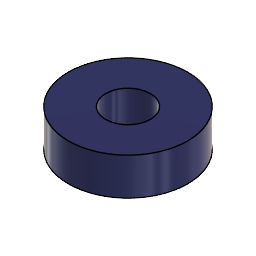
Asembly (Autodesk Fusion 360 archive; units mm, degrees)
design "Guolis 32-20-10"
Autodesk Fusion 360 part; units mm, degrees
sketch "Sketch1" plane through (0, 0, 0) normal (0, 0, 1) x (1, 0, 0)
  circle A0 centre (0, 0) radius 16
  circle A1 centre (0, 0) radius 6
  dimension "d1" = 32
  dimension "d2" = 12
  constraint coincident A0.centre A1.centre
  measures "d1" diameter of A0
  measures "d2" diameter of A1
extrude "Extrude1" add sketch "Sketch1" along normal blind 10

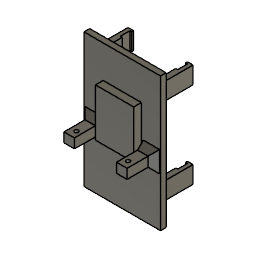
design "Wrist2"
Autodesk Fusion 360 part; units mm, degrees
sketch "Sketch1" plane through (0, 0, 0) normal (0, 1, 0) x (1, 0, 0)
  line L0 (-20, -35) -> (20, -35)
  line L1 (20, -35) -> (20, 35)
  line L2 (20, 35) -> (-20, 35)
  line L3 (-20, 35) -> (-20, -35)
  line L4 (-14.65, -4.5) -> (-12.65, -4.5)
  line L5 (-12.65, -4.5) -> (-12.65, 4.5)
  line L6 (-12.65, 4.5) -> (-14.65, 4.5)
  line L7 (-14.65, 4.5) -> (-14.65, -4.5)
  line L8 (12.65, -4.5) -> (14.65, -4.5)
  line L9 (14.65, -4.5) -> (14.65, 4.5)
  line L10 (14.65, 4.5) -> (12.65, 4.5)
  line L11 (12.65, 4.5) -> (12.65, -4.5)
  line L12 (-12.65, -4.5) -> (-11.65, -4.5)
  line L13 (-11.65, -4.5) -> (-11.65, 4.5)
  line L14 (-11.65, 4.5) -> (-12.65, 4.5)
  line L15 (-12.65, 4.5) -> (-12.65, -4.5)
  line L16 (12.65, -4.5) -> (11.65, -4.5)
  line L17 (11.65, -4.5) -> (11.65, 4.5)
  line L18 (11.65, 4.5) -> (12.65, 4.5)
  line L19 (12.65, 4.5) -> (12.65, -4.5)
  circle A0 centre (0, 0) radius 5
  line L20 (14, 16.5) -> (14, 25.5)
  line L21 (15, 16.5) -> (14, 16.5)
  line L22 (17, 16.5) -> (17, 25.5)
  line L23 (15, 25.5) -> (15, 16.5)
  line L24 (15, 16.5) -> (17, 16.5)
  line L25 (15, 25.5) -> (15, 16.5)
  line L26 (15, -19.5) -> (15, -28.5)
  line L27 (15, -19.5) -> (15, -28.5)
  line L28 (15, -28.5) -> (17, -28.5)
  line L29 (14, -28.5) -> (14, -19.5)
  line L30 (15, -28.5) -> (14, -28.5)
  line L31 (17, -28.5) -> (17, -19.5)
  line L32 (-15, -28.5) -> (-15, -19.5)
  line L33 (-17, -19.5) -> (-17, -28.5)
  line L34 (-15, -28.5) -> (-14, -28.5)
  line L35 (-14, -28.5) -> (-14, -19.5)
  line L36 (-15, -19.5) -> (-17, -19.5)
  line L37 (-15, -19.5) -> (-15, -28.5)
  line L38 (-14, -19.5) -> (-15, -19.5)
  line L39 (-17, -28.5) -> (-15, -28.5)
  line L40 (-15, 16.5) -> (-15, 25.5)
  line L41 (-17, 25.5) -> (-17, 16.5)
  line L42 (-15, 16.5) -> (-14, 16.5)
  line L43 (-14, 16.5) -> (-14, 25.5)
  line L44 (-15, 25.5) -> (-17, 25.5)
  line L45 (-15, 25.5) -> (-15, 16.5)
  line L46 (-14, 25.5) -> (-15, 25.5)
  line L47 (-17, 16.5) -> (-15, 16.5)
  line L48 (17, 25.5) -> (14, 25.5)
  line L49 (17, -19.5) -> (14, -19.5)
  line L50 (12.65, 1.5) -> (14.65, 1.5)
  line L51 (-14.65, 1.5) -> (-12.65, 1.5)
  line L52 (-10, -18) -> (10, -18)
  line L53 (10, -18) -> (10, 7)
  line L54 (10, 7) -> (-10, 7)
  line L55 (-10, 7) -> (-10, -18)
  line L56 (16.5, 1.5) -> (10.5, 1.5)
  line L57 (10.5, 1.5) -> (10.5, 6.5)
  line L58 (10.5, 6.5) -> (16.5, 6.5)
  line L59 (16.5, 6.5) -> (16.5, 1.5)
  line L60 (-10.5, 1.5) -> (-16.5, 1.5)
  line L61 (-16.5, 1.5) -> (-16.5, 6.5)
  line L62 (-16.5, 6.5) -> (-10.5, 6.5)
  line L63 (-10.5, 6.5) -> (-10.5, 1.5)
  dimension "d1" = 40
  dimension "d2" = 70
  dimension "d3" = 20
  dimension "d4" = 35
  dimension "d5" = 9
  dimension "d6" = 2
  dimension "d7" = 4.5
  dimension "d8" = 12.65
  dimension "d9" = 2
  dimension "d10" = 9
  dimension "d11" = 12.65
  dimension "d12" = 4.5
  dimension "d13" = 1
  dimension "d14" = 9
  dimension "d15" = 1
  dimension "d16" = 9
  dimension "d17" = 10
  dimension "d18" = 2
  dimension "d19" = 9
  dimension "d20" = 1
  dimension "d21" = 9
  dimension "d22" = 2
  dimension "d23" = 9
  dimension "d24" = 1
  dimension "d25" = 9
  dimension "d26" = 9
  dimension "d27" = 2
  dimension "d28" = 1
  dimension "d29" = 9
  dimension "d30" = 9
  dimension "d31" = 2
  dimension "d32" = 1
  dimension "d33" = 9
  dimension "d40" = 3
  dimension "d41" = 3
  dimension "d58" = 20
  dimension "d59" = 25
  dimension "d60" = 10
  dimension "d61" = 18
  dimension "d64" = 6
  dimension "d65" = 5
  dimension "d66" = 2.15
  dimension "d67" = 2.15
  dimension "d79" = 3
  dimension "d80" = 3
  dimension "d81" = 3
  dimension "d82" = 3
  constraint horizontal L0
  constraint vertical L1
  constraint horizontal L2
  constraint vertical L3
  constraint horizontal L4
  constraint vertical L5
  constraint horizontal L6
  constraint vertical L7
  constraint horizontal L8
  constraint vertical L9
  constraint horizontal L10
  constraint vertical L11
  constraint horizontal L12
  constraint vertical L13
  constraint horizontal L14
  constraint vertical L15
  constraint horizontal L16
  constraint vertical L17
  constraint horizontal L18
  constraint vertical L19
  constraint coincident A0.centre origin
  constraint horizontal L24
  constraint vertical L22
  constraint vertical L25
  constraint horizontal L21
  constraint vertical L20
  constraint vertical L23
  constraint horizontal L28
  constraint vertical L31
  constraint vertical L27
  constraint horizontal L30
  constraint vertical L29
  constraint vertical L26
  constraint horizontal L39
  constraint vertical L32
  constraint horizontal L36
  constraint vertical L33
  constraint horizontal L34
  constraint vertical L35
  constraint horizontal L38
  constraint vertical L37
  constraint horizontal L47
  constraint vertical L40
  constraint horizontal L44
  constraint vertical L41
  constraint horizontal L42
  constraint vertical L43
  constraint horizontal L46
  constraint vertical L45
  constraint perpendicular L20 L48
  constraint perpendicular L29 L49
  constraint coincident L11 L50.start
  constraint coincident L9 L50.end
  constraint perpendicular L9 L50
  constraint coincident L7 L51.start
  constraint coincident L5 L51.end
  constraint perpendicular L5 L51
  constraint horizontal L52
  constraint vertical L53
  constraint horizontal L54
  constraint vertical L55
  constraint horizontal L56
  constraint vertical L57
  constraint horizontal L58
  constraint vertical L59
  constraint horizontal L60
  constraint vertical L61
  constraint horizontal L62
  constraint vertical L63
  measures "d1" distance of L0.start L0.end
  measures "d2" distance of L0.start L2.end
  measures "d3" horizontal distance of A0.centre L0.start
  measures "d4" vertical distance of A0.centre L0.start
  measures "d5" distance of L4.start L6.end
  measures "d6" distance of L5.end L6.end
  measures "d7" vertical distance of A0.centre L4.end
  measures "d8" distance of A0.centre L5
  measures "d9" distance of L8.start L8.end
  measures "d10" distance of L8.start L10.end
  measures "d11" distance of A0.centre L11
  measures "d12" vertical distance of A0.centre L10.end
  measures "d13" distance of L4.end L12.end
  measures "d14" distance of L4.end L5.end
  measures "d15" distance of L8.start L16.end
  measures "d16" distance of L8.start L10.end
  measures "d17" diameter of A0
  measures "d18" distance of L22.start L21.start
  measures "d19" distance of L21.start L23.start
  measures "d20" distance of L21.start L20.start
  measures "d21" distance of L23.start L21.start
  measures "d22" distance of L28.end L26.end
  measures "d23" distance of L26.start L26.end
  measures "d24" distance of L26.end L29.start
  measures "d25" distance of L26.end L26.start
  measures "d26" distance of L33.end L33.start
  measures "d27" distance of L32.end L33.start
  measures "d28" distance of L32.start L34.end
  measures "d29" distance of L32.start L32.end
  measures "d30" distance of L41.end L41.start
  measures "d31" distance of L40.end L41.start
  measures "d32" distance of L40.start L42.end
  measures "d33" distance of L40.start L40.end
  measures "d40" distance of L10.end L50.start
  measures "d41" distance of L6.end L51.start
  measures "d58" distance of L52.start L52.end
  measures "d59" distance of L52.start L54.end
  measures "d60" distance of A0.centre L55
  measures "d61" distance of A0.centre L52
  measures "d64" distance of L60.start L60.end
  measures "d65" distance of L60.start L62.end
  measures "d66" distance of L19 L57
  measures "d67" distance of L5 L63
  measures "d79" distance of L1 L31
  measures "d80" distance of L3 L33
  measures "d81" distance of L1 L22
  measures "d82" distance of L3 L41
extrude "Extrude1" add sketch "Sketch1" along normal blind 3 contours L0 L1 L2 L3 | L4 L5 L7 L15 L51 L60 | L5 L12 L13 L15 L60 | L6 L7 L13 L14 L60 L61 L62 L63 | L5 L6 L7 L15 L51 L60 | L5 L13 L14 L15 L60 | L8 L9 L11 L19 L50 L56 | L11 L16 L17 L19 L56 | L11 L17 L18 L19 L56 | L9 L10 L11 L19 L50 L56 | L9 L10 L17 L18 L56 L57 L58 L59 | A0 | L20 L21 L23 L25 L48 | L22 L23 L24 L25 L48 | L26 L27 L28 L31 L49 | L26 L27 L29 L30 L49 | L32 L33 L36 L37 L39 | L32 L34 L35 L37 L38 | L40 L41 L44 L45 L47 | L40 L42 L43 L45 L46 | L52 L53 L54 L55
extrude "Extrude2" add sketch "Sketch1" against normal blind 14 contours L6 L7 L13 L14 L60 L61 L62 L63 | L5 L6 L7 L15 L51 L60 | L5 L13 L14 L15 L60 | L11 L17 L18 L19 L56 | L9 L10 L11 L19 L50 L56 | L9 L10 L17 L18 L56 L57 L58 L59
extrude "Extrude4" add sketch "Sketch1" along normal blind 20 contours L20 L21 L23 L25 L48 | L22 L23 L24 L25 L48 | L26 L27 L28 L31 L49 | L26 L27 L29 L30 L49 | L32 L33 L36 L37 L39 | L32 L34 L35 L37 L38 | L40 L41 L44 L45 L47 | L40 L42 L43 L45 L46
extrude "Extrude5" cut sketch "Sketch1" along normal blind 19 contours L20 L21 L23 L25 L48 | L26 L27 L29 L30 L49 | L32 L34 L35 L37 L38 | L40 L42 L43 L45 L46
extrude "Extrude6" add sketch "Sketch1" along normal blind 14 contours L20 L21 L23 L25 L48 | L26 L27 L29 L30 L49 | L32 L34 L35 L37 L38 | L40 L42 L43 L45 L46
chamfer "Chamfer3" distance 2 angle 45 12 edges at (-15.5, 3, -16.5) (-17, 3, 24) (-17, 3, -21) (-15.5, 3, -25.5) (15.5, 3, -25.5) (17, 3, -21) (15.5, 3, -16.5) (15.5, 3, 19.5) (17, 3, 24) (15.5, 3, 28.5) (-15.5, 3, 28.5) (-15.5, 3, 19.5)
extrude "Extrude7" add sketch "Sketch1" against normal blind 4 contours A0 | L52 L53 L54 L55
sketch "Sketch2" plane through (0, 0, -1.5) normal (0, 0, 1) x (-1, 0, 0)
  line L0 (10.5, 0) -> (16.5, 0)
  line L1 (16.5, 0) -> (16.5, 14)
  line L2 (16.5, 14) -> (10.5, 14)
  line L3 (10.5, 14) -> (10.5, 0)
  circle A0 centre (13.5, 10.39) radius 1
  circle A1 centre (-13.5, 10.39) radius 1
  line L4 (-10.5, 0) -> (-10.5, 14)
  line L5 (20, 0) -> (-20, 0)
  dimension "d68" = 2
  dimension "d70" = 10.39
  dimension "d71" = 3
  dimension "d72" = 2
  dimension "d73" = 3
  dimension "d74" = 10.39
  measures "d68" diameter of A0
  measures "d70" distance of L0 A0.centre
  measures "d71" distance of L3 A0.centre
  measures "d72" diameter of A1
  measures "d73" distance of A1.centre L4
  measures "d74" distance of A1.centre L5
extrude "Extrude8" cut sketch "Sketch2" against normal blind 9 contours A0 | A1
chamfer "Chamfer4" distance 3 angle 45 6 edges at (16.5, 0, -4) (13.5, 0, -1.5) (13.5, 0, -6.5) (-13.5, 0, -6.5) (-16.5, 0, -4) (-13.5, 0, -1.5)
move_face "OffsetFaces1" offset -0.5 2 faces at (10.5, -6.6667, -3.1667) (-10.5, -10.3333, -3.1667)

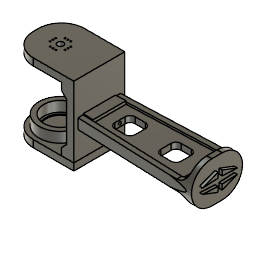
design "Arm2"
Autodesk Fusion 360 part; units mm, degrees
sketch "Sketch1" plane through (0, 0, 0) normal (0, 0, 1) x (1, 0, 0)
  circle A0 centre (-7.25, 0) radius 0.75
  line L0 (-4.3749, -7.25) -> (5.5, -7.25) construction
  circle A1 centre (0, -7.25) radius 0.75
  line L1 (7.25, -4) -> (7.25, 4) construction
  circle A2 centre (2.75, -7.25) radius 0.75
  circle A3 centre (-7.25, 2.75) radius 0.75
  circle A4 centre (7.25, 2.75) radius 0.75
  circle A5 centre (-7.25, -2.75) radius 0.75
  circle A6 centre (7.25, 0) radius 0.75
  circle A7 centre (0, 7.25) radius 0.75
  circle A8 centre (2.75, 7.25) radius 0.75
  line L2 (-7.25, -4.0817) -> (-7.25, 3.6702) construction
  circle A9 centre (-2.75, -7.25) radius 0.75
  circle A10 centre (-2.75, 7.25) radius 0.75
  line L3 (4.1, 7.25) -> (-3.9, 7.25) construction
  circle A11 centre (7.25, -2.75) radius 0.75
  circle A12 centre (0, 0) radius 15
  circle A13 centre (0, 0) radius 20
  line L4 (130, 25) -> (130, -25)
  line L5 (130, 25) -> (-0.7664, 19.9853)
  line L6 (130, -25) -> (-0.7664, -19.9853)
  line L7 (130, -19.9963) -> (-0.5748, -14.989)
  line L8 (-0.5748, 14.989) -> (130, 19.9963)
  circle A14 centre (0, 0) radius 3
  line L9 (105, -10) -> (85, -10)
  line L10 (85, -10) -> (85, 10)
  line L11 (85, 10) -> (105, 10)
  line L12 (105, 10) -> (105, -10)
  line L13 (60, -10) -> (40, -10)
  line L14 (40, 10) -> (60, 10)
  line L15 (40, -10) -> (40, 10)
  line L16 (60, 10) -> (60, -10)
  line L17 (19.8726, 20.7768) -> (19.8726, -20.7768)
  line L18 (29.8726, -16.1566) -> (29.8726, 16.1566)
  dimension "d1" = 1.5
  dimension "d2" = 7.25
  dimension "d3" = 1.5
  dimension "d4" = 1.5
  dimension "d5" = 1.5
  dimension "d6" = 1.5
  dimension "d7" = 1.5
  dimension "d8" = 1.5
  dimension "d9" = 1.5
  dimension "d10" = 1.5
  dimension "d11" = 1.5
  dimension "d12" = 1.5
  dimension "d13" = 1.5
  dimension "d14" = 2.75
  dimension "d15" = 2.75
  dimension "d16" = 2.75
  dimension "d17" = 2.75
  dimension "d18" = 2.75
  dimension "d19" = 7.25
  dimension "d20" = 2.75
  dimension "d21" = 2.75
  dimension "d22" = 2.75
  dimension "d23" = 7.25
  dimension "d24" = 2.75
  dimension "d25" = 2.75
  dimension "d26" = 2.75
  dimension "d27" = 7.25
  dimension "d28" = 2.75
  dimension "d30" = 30
  dimension "d31" = 40
  dimension "d32" = 50
  dimension "d33" = 25
  dimension "d34" = 130
  dimension "d44" = 6
  dimension "d51" = 20
  dimension "d52" = 20
  dimension "d53" = 10
  dimension "d54" = 85
  dimension "d55" = 20
  dimension "d56" = 20
  dimension "d57" = 40
  dimension "d58" = 10
  dimension "d190" = 10
  constraint coincident A12.centre A13.centre
  constraint vertical L2
  constraint coincident A3.centre L2
  constraint coincident A5.centre L2
  constraint horizontal L0
  constraint coincident A0.centre L2
  constraint coincident A2.centre L0
  constraint coincident A1.centre L0
  constraint coincident A9.centre L0
  constraint vertical L1
  constraint coincident A11.centre L1
  constraint coincident A6.centre L1
  constraint coincident A4.centre L1
  constraint horizontal L3
  constraint coincident A8.centre L3
  constraint coincident A7.centre L3
  constraint coincident A10.centre L3
  constraint concentric A12 A13
  constraint vertical L4
  constraint coincident A13 L6.end
  constraint tangent A13 L6
  constraint coincident L4 L7.start
  constraint coincident A12 L7.end
  constraint tangent A12 L7
  constraint coincident A12 L8.start
  constraint coincident L4 L8.end
  constraint tangent A12 L8
  constraint parallel L5 L8
  constraint parallel L6 L7
  constraint coincident A13 L5.end
  constraint tangent A13 L5
  constraint horizontal L9
  constraint vertical L10
  constraint horizontal L11
  constraint vertical L12
  constraint horizontal L13
  constraint vertical L15
  constraint horizontal L14
  constraint vertical L16
  constraint coincident L5 L17.start
  constraint coincident L6 L17.end
  constraint vertical L17
  constraint coincident L7 L18.start
  constraint coincident L8 L18.end
  constraint vertical L18
  measures "d1" diameter of A0
  measures "d2" distance of A12.centre A0.centre
  measures "d3" diameter of A3
  measures "d4" diameter of A5
  measures "d5" diameter of A1
  measures "d6" diameter of A2
  measures "d7" diameter of A9
  measures "d8" diameter of A7
  measures "d9" diameter of A10
  measures "d10" diameter of A8
  measures "d11" diameter of A6
  measures "d12" diameter of A11
  measures "d13" diameter of A4
  measures "d14" distance of A0.centre A5.centre
  measures "d15" distance of A0.centre A3.centre
  measures "d16" vertical distance of A3.centre A12.centre
  measures "d17" distance of A2.centre A1.centre
  measures "d18" distance of A9.centre A1.centre
  measures "d19" distance of A1.centre A12.centre
  measures "d20" horizontal distance of A9.centre A12.centre
  measures "d21" distance of A6.centre A11.centre
  measures "d22" distance of A4.centre A6.centre
  measures "d23" distance of A6.centre A12.centre
  measures "d24" vertical distance of A11.centre A12.centre
  measures "d25" distance of A7.centre A10.centre
  measures "d26" distance of A7.centre A8.centre
  measures "d27" distance of A7.centre A12.centre
  measures "d28" horizontal distance of A8.centre A12.centre
  measures "d30" diameter of A12
  measures "d31" diameter of A13
  measures "d32" distance of L4.start L4.end
  measures "d33" vertical distance of A12.centre L4.start
  measures "d34" distance of A12.centre L4
  measures "d44" diameter of A14
  measures "d51" distance of L9.start L9.end
  measures "d52" distance of L9.start L11.end
  measures "d53" vertical distance of A12.centre L9.end
  measures "d54" distance of A12.centre L10
  measures "d55" distance of L13.end L13.start
  measures "d56" distance of L14.end L13.start
  measures "d57" distance of A12.centre L15
  measures "d58" vertical distance of A12.centre L13.end
  measures "d190" distance of L17 L18
extrude "Extrude1" add sketch "Sketch1" along normal mid plane 6 contours A13 L7 L8 L17 L18 | L4 L7 L8 L18 makes body 1
extrude "Extrude2" add sketch "Sketch1" along normal mid plane 10 contours A13 L17 | L4 L5 L8 L17 | L4 L6 L7 L17 bodies 1
sketch "Sketch3" plane through (130, 0, 0) normal (1, 0, 0) x (0, 1, 0)
  line L0 (19.9963, 3) -> (-19.9963, 3)
  line L1 (-19.9963, 3) -> (-19.9963, 5)
  line L2 (-19.9963, 5) -> (-25, 5)
  line L3 (-25, 5) -> (-25, -5)
  line L4 (-25, -5) -> (-19.9963, -5)
  line L5 (-19.9963, -5) -> (-19.9963, -3)
  line L6 (-19.9963, -3) -> (19.9963, -3)
  line L7 (19.9963, -3) -> (19.9963, -5)
  line L8 (19.9963, -5) -> (25, -5)
  line L9 (25, -5) -> (25, 5)
  line L10 (25, 5) -> (19.9963, 5)
  line L11 (19.9963, 5) -> (19.9963, 3)
  line L12 (-25, 20) -> (25, 20)
  line L13 (25, 20) -> (25, -20)
  line L14 (25, -20) -> (-25, -20)
  line L15 (-25, -20) -> (-25, 20)
  circle A0 centre (14.5, 0) radius 0.5
  circle A1 centre (-14.5, 0) radius 0.5
  dimension "d45" = 50
  dimension "d46" = 40
  dimension "d47" = 25
  dimension "d48" = 20
  dimension "d63" = 1
  dimension "d64" = 14.5
  dimension "d65" = 1
  dimension "d66" = 14.5
  constraint horizontal L12
  constraint vertical L13
  constraint horizontal L14
  constraint vertical L15
  measures "d45" distance of L12.start L12.end
  measures "d46" distance of L12.start L14.end
  measures "d47" horizontal distance of origin L12.start
  measures "d48" vertical distance of origin L12.start
  measures "d63" diameter of A0
  measures "d64" distance of origin A0.centre
  measures "d65" diameter of A1
  measures "d66" distance of origin A1.centre
extrude "Extrude4" add sketch "Sketch3" along normal blind 5 bodies 1
fillet "Fillet1" radius 5 8 edges at (40, 10, 0) (60, 10, 0) (60, -10, 0) (40, -10, 0) (85, -10, 0) (105, 10, 0) (105, -10, 0) (85, 10, 0) on bodies 1
fillet "Fillet2" radius 10 10 edges at (130, 0, 3) (130, -22.4982, 5) (130, 22.4982, 5) (130, 19.9963, 4) (130, -19.9963, 4) (130, 22.4982, -5) (130, 19.9963, -4) (130, 0, -3) (130, -19.9963, -4) (130, -22.4982, -5) on bodies 1
sketch "Sketch4" plane through (135, 0, 0) normal (1, 0, 0) x (0, 1, 0)
  circle A0 centre (-14.5, 0) radius 0.5
  circle A1 centre (14.5, 0) radius 0.5
  line L0 (-25, -20) -> (25, -20)
  line L1 (25, -20) -> (25, 20)
  line L2 (25, 20) -> (-25, 20)
  line L3 (-25, 20) -> (-25, -20)
  line L4 (-2, 8.5) -> (-2, 3.5)
  line L5 (-2, 3.5) -> (-16.9794, 2.715)
  line L6 (-16.9794, 2.715) -> (-2, 8.5)
  line L7 (2, 8.5) -> (2, 3.5)
  line L8 (16.9794, 2.715) -> (2, 8.5)
  line L9 (2, 3.5) -> (16.9794, 2.715)
  line L10 (-2, -3.5) -> (-2, -8.5)
  line L11 (-2, -8.5) -> (-16.9794, -2.715)
  line L12 (-16.9794, -2.715) -> (-2, -3.5)
  line L13 (2, -3.5) -> (2, -8.5)
  line L14 (2, -8.5) -> (16.9794, -2.715)
  line L15 (16.9794, -2.715) -> (2, -3.5)
  circle A2 centre (0, 0) radius 2
  dimension "d67" = 5
  dimension "d68" = 15
  dimension "d69" = 3.5
  dimension "d70" = 2
  dimension "d71" = 93
  dimension "d82" = 5
  dimension "d83" = 15
  dimension "d84" = 93
  dimension "d85" = 3.5
  dimension "d86" = 2
  dimension "d87" = 2
  dimension "d95" = 15
  dimension "d96" = 5
  dimension "d97" = 2
  dimension "d98" = 93
  dimension "d99" = 3.5
  dimension "d100" = 93
  dimension "d101" = 5
  dimension "d103" = 15
  dimension "d104" = 3.5
  dimension "d105" = 2
  dimension "d110" = 4
  constraint vertical L4
  constraint vertical L10
  constraint vertical L13
  constraint coincident A2.centre origin
  measures "d67" distance of L4.start L4.end
  measures "d68" distance of L4.end L5.end
  measures "d69" vertical distance of A2.centre L4.end
  measures "d70" distance of A2.centre L4
  measures "d71" angle of L4 L5
  measures "d82" distance of L7.start L7.end
  measures "d83" distance of L8.start L7.end
  measures "d84" angle of L7 L9
  measures "d85" vertical distance of A2.centre L7.end
  measures "d86" horizontal distance of A2.centre L7.start
  measures "d87" horizontal distance of A2.centre L7.end
  measures "d95" distance of L10.start L11.end
  measures "d96" distance of L10.start L10.end
  measures "d97" horizontal distance of A2.centre L10.end
  measures "d98" angle of L10 L12
  measures "d99" vertical distance of A2.centre L10.start
  measures "d100" angle of L13 L15
  measures "d101" distance of L13.start L13.end
  measures "d103" distance of L13.start L14.end
  measures "d104" vertical distance of A2.centre L13.start
  measures "d105" horizontal distance of A2.centre L13.end
  measures "d110" diameter of A2
extrude "Extrude5" add sketch "Sketch4" along normal blind 3 contours L4 L5 L6 | L7 L8 L9 | L10 L11 L12 | L13 L14 L15 bodies 1
fillet "Fillet3" radius 20 4 edges at (132.5, -25, 20) (132.5, 25, 20) (132.5, 25, -20) (132.5, -25, -20) on bodies 1
sketch "Sketch5" plane through (19.8726, 0, 0) normal (-1, 0, 0) x (0, -1, 0)
  line L0 (-2.2536, 3) -> (-15.7731, 3)
  line L1 (-15.7731, 3) -> (-15.7731, 5)
  line L2 (-15.7731, 5) -> (-20.7768, 5)
  line L3 (-20.7768, 5) -> (-20.7768, -5)
  line L4 (-20.7768, -5) -> (-15.7731, -5)
  line L5 (-15.7731, -5) -> (-15.7731, -3)
  line L6 (-15.7731, -3) -> (-2.2536, -3)
  line L7 (-2.2536, -3) -> (-2.2536, -5)
  line L8 (-2.2536, -5) -> (2.2536, -5)
  line L9 (2.2536, -5) -> (2.2536, -3)
  line L10 (2.2536, -3) -> (15.7731, -3)
  line L11 (15.7731, -3) -> (15.7731, -5)
  line L12 (15.7731, -5) -> (20.7768, -5)
  line L13 (20.7768, -5) -> (20.7768, 5)
  line L14 (20.7768, 5) -> (15.7731, 5)
  line L15 (15.7731, 5) -> (15.7731, 3)
  line L16 (15.7731, 3) -> (2.2536, 3)
  line L17 (2.2536, 3) -> (2.2536, 5)
  line L18 (2.2536, 5) -> (-2.2536, 5)
  line L19 (-2.2536, 5) -> (-2.2536, 3)
  line L20 (25, 38.1) -> (-25, 38.1)
  line L21 (-25, 38.1) -> (-25, -38.1)
  line L22 (-25, -38.1) -> (25, -38.1)
  line L23 (25, -38.1) -> (25, 38.1)
  line L24 (25, -31.1) -> (-25, -31.1)
  line L25 (25, 31.1) -> (-25, 31.1)
  line L26 (-25, -24.1) -> (25, -24.1)
  line L27 (-25, 24.1) -> (25, 24.1)
  dimension "d111" = 76.2
  dimension "d112" = 50
  dimension "d113" = 38.1
  dimension "d114" = 7
  dimension "d115" = 25
  dimension "d116" = 7
  dimension "d155" = 7
  dimension "d163" = 7
  constraint horizontal L20
  constraint vertical L21
  constraint horizontal L22
  constraint vertical L23
  constraint coincident L21 L24.end
  constraint perpendicular L21 L24
  constraint coincident L23 L24.start
  constraint coincident L23 L25.start
  constraint coincident L21 L25.end
  constraint perpendicular L21 L25
  constraint coincident L21 L26.start
  constraint coincident L23 L26.end
  constraint perpendicular L23 L26
  constraint coincident L21 L27.start
  constraint coincident L23 L27.end
  constraint perpendicular L23 L27
  measures "d111" distance of L20 L22
  measures "d112" distance of L21.end L22.end
  measures "d113" vertical distance of origin L22.end
  measures "d114" distance of L22.end L24.start
  measures "d115" horizontal distance of origin L22.end
  measures "d116" distance of L20.start L25.start
  measures "d155" distance of L24 L26
  measures "d163" distance of L25 L27
extrude "Extrude6" add sketch "Sketch5" along normal blind 7 separate body contours L0 L1 L2 L3 L4 L5 L6 L7 L8 L9 L10 L11 L12 L13 L14 L15 L16 L17 L18 L19 | L20 L21 L23 L25 | L21 L23 L25 L27 | L21 L23 L26 L27 | L21 L23 L24 L26 makes body 2
extrude "Extrude7" add sketch "Sketch5" along normal blind 62 contours L20 L21 L23 L25 bodies 2
extrude "Extrude1'" add sketch "Sketch5" along normal blind 62 separate body contours L21 L22 L23 L24 makes body 3 in component "Component"
sketch "Sketch6" plane through (0, 0, 31.1) normal (0, 0, -1) x (1, 0, 0)
  line L0 (12.8726, -25) -> (12.8726, 25)
  line L1 (12.8726, 25) -> (-42.1274, 25)
  line L2 (-42.1274, 25) -> (-42.1274, -25)
  line L3 (-42.1274, -25) -> (12.8726, -25)
  circle A0 centre (-18.1274, -7.25) radius 0.75
  circle A1 centre (-20.8774, -7.25) radius 0.75
  circle A2 centre (-25.3774, 0) radius 0.75
  circle A3 centre (-25.3774, 2.75) radius 0.75
  circle A4 centre (-10.8774, -2.75) radius 0.75
  circle A5 centre (-25.3774, -2.75) radius 0.75
  line L4 (-10.9951, -7.25) -> (-1.1202, -7.25) construction
  line L5 (-25.3774, -4.5317) -> (-25.3774, 3.2202) construction
  circle A6 centre (-15.3774, -7.25) radius 0.75
  line L6 (-10.8774, -4.45) -> (-10.8774, 3.55) construction
  circle A7 centre (-20.8774, 7.25) radius 0.75
  line L7 (-2.5202, 7.25) -> (-10.5202, 7.25) construction
  circle A8 centre (-10.8774, 2.75) radius 0.75
  circle A9 centre (-18.1274, 0) radius 3
  circle A10 centre (-18.1274, 7.25) radius 0.75
  circle A11 centre (-10.8774, 0) radius 0.75
  circle A12 centre (-15.3774, 7.25) radius 0.75
  point P0 (-18.1274, 0)
  point P1 (-18.1274, 0)
  point P2 (-18.1274, 0)
  point P3 (-18.1274, 0)
  point P4 (-18.1274, 0)
  point P5 (-18.1274, 0)
  point P6 (-18.1274, 0)
  point P7 (-18.1274, 0)
  dimension "d123" = 6
  dimension "d124" = 1.5
  dimension "d125" = 7.25
  dimension "d126" = 1.5
  dimension "d127" = 1.5
  dimension "d128" = 1.5
  dimension "d129" = 1.5
  dimension "d130" = 1.5
  dimension "d131" = 1.5
  dimension "d132" = 1.5
  dimension "d133" = 1.5
  dimension "d134" = 1.5
  dimension "d135" = 1.5
  dimension "d136" = 1.5
  dimension "d137" = 2.75
  dimension "d138" = 2.75
  dimension "d139" = 2.75
  dimension "d140" = 2.75
  dimension "d141" = 2.75
  dimension "d142" = 7.25
  dimension "d143" = 2.75
  dimension "d144" = 2.75
  dimension "d145" = 2.75
  dimension "d146" = 7.25
  dimension "d147" = 2.75
  dimension "d148" = 2.75
  dimension "d149" = 2.75
  dimension "d150" = 7.25
  dimension "d151" = 2.75
  dimension "d153" = 25
  dimension "d154" = 24
  constraint coincident P7 P4
  constraint coincident P5 P4
  constraint coincident P7 P6
  constraint vertical L5
  constraint coincident A3.centre L5
  constraint coincident A5.centre L5
  constraint horizontal L4
  constraint coincident A2.centre L5
  constraint coincident A6.centre L4
  constraint coincident A0.centre L4
  constraint coincident A1.centre L4
  constraint vertical L6
  constraint coincident A4.centre L6
  constraint coincident A11.centre L6
  constraint coincident A8.centre L6
  constraint horizontal L7
  constraint coincident A12.centre L7
  constraint coincident A10.centre L7
  constraint coincident A7.centre L7
  measures "d123" diameter of A9
  measures "d124" diameter of A2
  measures "d125" distance of P7 A2.centre
  measures "d126" diameter of A3
  measures "d127" diameter of A5
  measures "d128" diameter of A0
  measures "d129" diameter of A6
  measures "d130" diameter of A1
  measures "d131" diameter of A10
  measures "d132" diameter of A7
  measures "d133" diameter of A12
  measures "d134" diameter of A11
  measures "d135" diameter of A4
  measures "d136" diameter of A8
  measures "d137" distance of A5.centre A2.centre
  measures "d138" distance of A3.centre A2.centre
  measures "d139" vertical distance of P7 A3.centre
  measures "d140" distance of A0.centre A6.centre
  measures "d141" distance of A0.centre A1.centre
  measures "d142" distance of A0.centre P7
  measures "d143" horizontal distance of P7 A1.centre
  measures "d144" distance of A11.centre A4.centre
  measures "d145" distance of A11.centre A8.centre
  measures "d146" distance of P7 A11.centre
  measures "d147" vertical distance of A4.centre P7
  measures "d148" distance of A7.centre A10.centre
  measures "d149" distance of A12.centre A10.centre
  measures "d150" distance of P7 A10.centre
  measures "d151" horizontal distance of P7 A12.centre
  measures "d153" distance of L1 P7
  measures "d154" distance of L2 P7
extrude "Extrude8" add sketch "Sketch5" along normal blind 12 contours L21 L23 L25 L27 | L21 L23 L24 L26 bodies 2
chamfer "Chamfer1" distance 5 angle 45 1 edges at (12.8726, 0, -24.1) on bodies 2
chamfer "Chamfer1" distance 5 angle 45 1 edges at (12.8726, 0, 24.1) on bodies 2
sketch "Sketch7" plane through (0, 0, -31.1) normal (0, 0, 1) x (-1, 0, 0)
  line L0 (-19.8726, 25) -> (-19.8726, -25)
  line L1 (-19.8726, -25) -> (42.1274, -25)
  line L2 (42.1274, -25) -> (42.1274, 25)
  line L3 (42.1274, 25) -> (-19.8726, 25)
  circle A0 centre (18.1274, 0) radius 16
  line L4 (42.1274, 25) -> (42.1274, -25)
  line L5 (42.1274, -25) -> (-12.8726, -25)
  circle A1 centre (18.1274, 0) radius 21
  circle A2 centre (18.1274, 0) radius 14
  dimension "d159" = 32
  dimension "d161" = 25
  dimension "d162" = 24
  dimension "d165" = 42
  dimension "d166" = 28
  constraint concentric A0 A1
  constraint concentric A0 A2
  measures "d159" diameter of A0
  measures "d161" distance of A0.centre L5
  measures "d162" distance of L2 A0.centre
  measures "d165" diameter of A1
  measures "d166" diameter of A2
extrude "Extrude2'" cut sketch "Sketch7" against normal blind 1 contours A2 bodies 3 in component "Component"
extrude "Extrude3" add sketch "Sketch7" along normal blind 10 contours A1 bodies 3 in component "Component"
sketch "Sketch8" plane through (0, 0, -38.1) normal (0, 0, -1) x (1, 0, 0)
  line L0 (19.8726, -25) -> (19.8726, 25)
  line L1 (19.8726, 25) -> (-42.1274, 25)
  line L2 (-42.1274, 25) -> (-42.1274, -25)
  line L3 (-42.1274, -25) -> (19.8726, -25)
  circle A0 centre (14.8726, -14.6969) radius 2
  circle A1 centre (11.8726, 0) radius 2
  circle A2 centre (14.8726, 14.6969) radius 2
  dimension "d171" = 4
  dimension "d172" = 4
  dimension "d173" = 4
  dimension "d174" = 15
  dimension "d175" = 15
  dimension "d176" = 5
  dimension "d177" = 5
  dimension "d178" = 25
  dimension "d179" = 8
  measures "d171" diameter of A0
  measures "d172" diameter of A1
  measures "d173" diameter of A2
  measures "d174" distance of A1.centre A2.centre
  measures "d175" distance of A0.centre A1.centre
  measures "d176" distance of L0 A0.centre
  measures "d177" distance of L0 A2.centre
  measures "d178" distance of L3 A1.centre
  measures "d179" distance of L0 A1.centre
extrude "Extrude9" cut sketch "Sketch8" against normal blind 18 contours A0 | A1 | A2 bodies 2
extrude "Extrude4'" cut sketch "Sketch8" against normal blind 18 contours A0 | A1 | A2 bodies 3 in component "Component"
extrude "Extrude10" cut sketch "Sketch6" against normal blind 11 contours A0 | A1 | A2 | A3 | A4 | A5 | A6 | A7 | A8 | A9 | A10 | A11 | A12 bodies 2
fillet "Fillet4" radius 22.5 2 edges at (-42.1274, -25, 34.6) (-42.1274, 25, 34.6) on bodies 2
fillet "Fillet1'" radius 22.5 2 edges at (-42.1274, -25, -34.6) (-42.1274, 25, -34.6) on bodies 3 in component "Component"
extrude "Extrude11" add sketch "Sketch1" along normal mid plane 12 contours A13 L7 L8 L17 L18 bodies 1
sketch "Sketch9" plane through (12.8726, 0, 0) normal (-1, 0, 0) x (0, -1, 0)
  line L0 (25, 19.1) -> (-25, 19.1)
  line L1 (-25, 19.1) -> (-25, -19.1)
  line L2 (-25, -19.1) -> (25, -19.1)
  line L3 (25, -19.1) -> (25, 19.1)
  circle A0 centre (-15, 0.0157) radius 1.5
  circle A1 centre (0, 0) radius 1.5
  circle A2 centre (15, 0.0157) radius 1.5
  dimension "d193" = 3
  dimension "d194" = 3
  dimension "d195" = 3
  dimension "d196" = 15
  dimension "d197" = 15
  constraint coincident A1.centre origin
  measures "d193" diameter of A0
  measures "d194" diameter of A1
  measures "d195" diameter of A2
  measures "d196" distance of A1.centre A2.centre
  measures "d197" distance of A1.centre A0.centre
extrude "Extrude12" cut sketch "Sketch9" against normal blind 28 contours A0 | A1 | A2 bodies 1 2
move_face "OffsetFaces1" offset -0.2 1 faces at (-34.1075, 0.7975, -24.4333) on bodies 3 in component "Component"
component "Component" placed x (1, 0, 0) y (0, 1, 0) z (0, 0, 1) at (0, 0, 0)
equation "d119 = 47 mm + 15 mm"
equation "d121 = 47 mm + 15 mm"
equation "d162 = 16 mm + 8 mm"

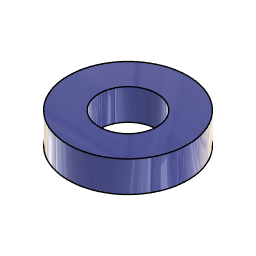
design "guolis-6206zz-30x62x16"
Autodesk Fusion 360 part; units mm, degrees
sketch "Sketch1" plane through (0, 0, 0) normal (0, 0, 1) x (1, 0, 0)
  circle A0 centre (0, 0) radius 15
  circle A1 centre (0, 0) radius 31
  dimension "d1" = 62
  dimension "d2" = 30
  constraint coincident A0.centre A1.centre
  measures "d1" diameter of A1
  measures "d2" diameter of A0
extrude "Extrude1" add sketch "Sketch1" along normal blind 16
